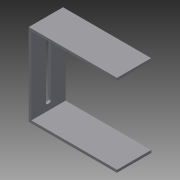
# Autodesk Inventor part: Fork x ver2
Saved by Autodesk Inventor 2015 (Build 190159000, 159)
## iProperties
Created: 2015-06-22
Part Number: Fork x ver2
Material: 一般
Document SubType Name: Modeling
Designer: kenta
Density: 1 g/cm^3
Appearance: 既定
Author: kenta
Autodesk Inventor part; units mm, degrees
ref_plane "YZ Plane" through (0, 0, 0) normal (1, 0, 0) x (0, 1, 0)
ref_plane "XZ Plane" through (0, 0, 0) normal (0, 1, 0) x (-1, 0, 0)
ref_plane "XY Plane" through (0, 0, 0) normal (0, 0, 1) x (1, 0, 0)
sketch "スケッチ1" plane through (0, 0, 0) normal (0, 0, 1) x (1, 0, 0)
  line L0 (-25, 10) -> (25, 10)
  line L1 (25, 10) -> (25, -10)
  line L2 (25, -10) -> (-25, -10)
  line L3 (-25, -10) -> (-25, 10)
  line L4 (-25, 10) -> (25, -10) construction
  line L5 (25, 10) -> (-25, -10) construction
  point P0 (0, 0)
  dimension "d0" = 50
  dimension "d1" = 20
  constraints: 12 end point, 2 midpoint, 2 parallel, 1 horizontal, 1 perpendicular
  measures "d0" distance of L1.end L2.end
  measures "d1" distance of L0.end L1.end
extrude "押し出し1" add sketch "スケッチ1" along normal blind 1.5
sketch "スケッチ2" plane through (-25, -10, 0) normal (-1, 0, 0) x (0, 0, 1)
  line L0 (0, 0) -> (48, 0)
  line L1 (48, 0) -> (48, 20)
  line L2 (48, 20) -> (0, 20)
  line L3 (0, 20) -> (0, 0)
  line L4 (0, 0) -> (0, 20) projected
  line L5 (0, 0) -> (1.5, 0) projected
  point P0 (0, 10)
  dimension "d4" = 48
  dimension "d5" = 20
  dimension "d6" = 0
  dimension "d7" = 0
  constraints: 8 end point, 2 parallel, 1 horizontal, 1 perpendicular
  measures "d4" distance of L2.end L1.end
  measures "d5" distance of L1.end L0.end
  measures "d6" distance between parallel lines of L4 L3
  measures "d7" distance between parallel lines of L5 L0
extrude "押し出し2" add sketch "スケッチ2" along normal blind 1.5
sketch "スケッチ4" plane through (-25, -10, 0) normal (1, 0, 0) x (0, 0, -1)
  line L0 (-48, 0) -> (-46.5, 0)
  line L1 (-46.5, 0) -> (-46.5, 20)
  line L2 (-46.5, 20) -> (-48, 20)
  line L3 (-48, 20) -> (-48, 0)
  point P0 (0, 10)
  dimension "d10" = 1.5
  constraints: 8 end point, 2 parallel, 1 horizontal, 1 perpendicular
  measures "d10" distance of L2.end L1.end
extrude "押し出し3" add sketch "スケッチ4" along normal blind 50
sketch "スケッチ5" plane through (-26.5, -10, 0) normal (-1, 0, 0) x (0, 0, 1)
  line L0 (5, 11.5) -> (43, 11.5)
  line L1 (43, 11.5) -> (43, 8.5)
  line L2 (43, 8.5) -> (5, 8.5)
  line L3 (5, 8.5) -> (5, 11.5)
  line L4 (48, 0) -> (48, 20) projected
  line L5 (48, 20) -> (0, 20) projected
  line L6 (0, 0) -> (48, 0) projected
  line L7 (0, 20) -> (0, 0) projected
  point P0 (0, 10)
  dimension "d13" = 3
  dimension "d14" = 38
  dimension "d15" = 5
  dimension "d16" = 8.5
  dimension "d17" = 8.5
  dimension "d18" = 5
  constraints: 8 end point, 2 parallel, 1 horizontal, 1 perpendicular
  measures "d13" distance of L0.end L1.end
  measures "d14" distance of L1.end L2.end
  measures "d15" distance between parallel lines of L4 L1
  measures "d16" distance between parallel lines of L5 L0
  measures "d17" distance between parallel lines of L2 L6
  measures "d18" distance between parallel lines of L3 L7
extrude "押し出し4" cut sketch "スケッチ5" against normal blind 3 contours L0 L1 L2 L3
fillet "フィレット1" radius 1 4 edges at (-25.75, -1.5, 43) (-25.75, 1.5, 43) (-25.75, -1.5, 5) (-25.75, 1.5, 5)
